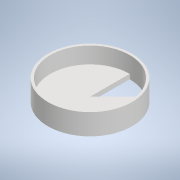
# Autodesk Inventor part: FeedWheelShell
Saved by Autodesk Inventor 2020 (Build 240168000, 168)
## iProperties
Created: 2020-03-05
Part Number: FeedWheelShell
Material: Generic
Document SubType Name: Modeling
Designer: jared.jones280
Density: 1 g/cm^3
Appearance: Default
Author: jared.jones280
Autodesk Inventor part; units mm, degrees
ref_plane "YZ Plane" through (0, 0, 0) normal (1, 0, 0) x (0, 1, 0)
ref_plane "XZ Plane" through (0, 0, 0) normal (0, 1, 0) x (-1, 0, 0)
ref_plane "XY Plane" through (0, 0, 0) normal (0, 0, 1) x (1, 0, 0)
sketch "Sketch1" plane through (0, 0, 0) normal (0, 1, 0) x (-1, 0, 0)
  circle A0 centre (0, 0) radius 57.15
  circle A1 centre (0, 0) radius 53.975
  dimension "d0" = 114.3
  dimension "d1" = 107.95
  constraints: 2 centre point, 2 coincident
  measures "d0" diameter of A0
  measures "d1" diameter of A1
extrude "Extrusion1" add sketch "Sketch1" along normal blind 28.575 contours A0 | A1
sketch "Sketch2" plane through (0, 28.575, 0) normal (0, 1, 0) x (1, 0, 0)
  circle A0 centre (0, 0) radius 53.975
  dimension "d4" = 107.95
  constraints: 1 centre point, 1 coincident
  measures "d4" diameter of A0
extrude "Extrusion2" cut sketch "Sketch2" against normal blind 22.225
sketch "Sketch3" plane through (0, 6.35, 0) normal (0, 1, 0) x (1, 0, 0)
  circle A0 centre (0, 0) radius 53.975 projected
  line L0 (0, 53.975) -> (0, 0)
  line L1 (0, 0) -> (53.975, 0)
  line L2 (0, 0) -> (40.4112, 40.4112)
  line L3 (0, 0) -> (57.15, 0) construction
  point P0 (38.1661, 38.1661)
  dimension "d7" = 57.15
  dimension "d8" = 45
  constraints: 8 end point, 2 point on circle, 1 equal length, 1 horizontal, 1 vertical
  measures "d7" distance of L0.end L2.end
  measures "d8" angle of L3 L2
extrude "Extrusion3" cut sketch "Sketch3" against normal blind 22.225 contours A0 L2 L0
fillet "Fillet1" radius 0.762 3 edges at (0, 3.175, 0) (0, 3.175, -53.975) (38.1661, 3.175, -38.1661)
body "Solid1"
